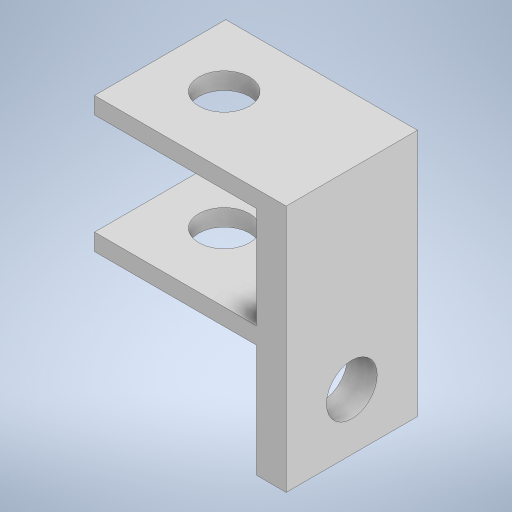
# Autodesk Inventor part: rodclamp1
Saved by Autodesk Inventor 2024.1 (Build 281209000, 209)
## iProperties
Created: 2024-01-24
Part Number: rodclamp1
Material: Generic
Document SubType Name: Modeling
Designer: udayk
Density: 1 g/cm^3
Appearance: Default
Author: udayk
Autodesk Inventor part; units mm, degrees
ref_plane "YZ Plane" through (0, 0, 0) normal (1, 0, 0) x (0, 1, 0)
ref_plane "XZ Plane" through (0, 0, 0) normal (0, 1, 0) x (-1, 0, 0)
ref_plane "XY Plane" through (0, 0, 0) normal (0, 0, 1) x (1, 0, 0)
sketch "Sketch1" plane through (0, 0, 0) normal (1, 0, 0) x (0, 1, 0)
  line L0 (0, 0) -> (12, 0)
  line L1 (12, 0) -> (12, -11.65)
  line L2 (12, -11.65) -> (0, -11.65)
  line L3 (0, -11.65) -> (0, 0)
  dimension "d0" = 12
  dimension "d1" = 11.65
  constraints: 8 end point, 2 parallel, 1 horizontal, 1 perpendicular
  measures "d0" distance of L1.end L2.end
  measures "d1" distance between parallel lines of L0 L2
extrude "Extrusion1" add sketch "Sketch1" along normal blind 17
sketch "Sketch3" plane through (0, 0, 0) normal (0, 0, 1) x (1, 0, 0)
  line L0 (-0.6451, 10.5) -> (14.3549, 10.5)
  line L1 (14.3549, 10.5) -> (14.3549, 1.5)
  line L2 (14.3549, 1.5) -> (-0.6451, 1.5)
  line L3 (-0.6451, 1.5) -> (-0.6451, 10.5)
  line L4 (17, 12) -> (17, 0) projected
  line L5 (0, 12) -> (17, 12) projected
  point P0 (0, 0)
  point P1 (10, 1.5)
  point P2 (10, 10.5)
  dimension "d7" = 9
  dimension "d8" = 15
  dimension "d10" = 1.5
  constraints: 8 end point, 2 parallel, 1 horizontal, 1 perpendicular
  measures "d7" distance between parallel lines of L2 L0
  measures "d8" distance between parallel lines of L3 L1
  measures "d10" distance between parallel lines of L5 L0
extrude "Extrusion2" cut sketch "Sketch3" against normal blind 14
sketch "Sketch5" plane through (0, 12, 0) normal (0, 1, 0) x (1, 0, 0)
  circle A0 centre (5.4549, 6.05) radius 2.25
  line L0 (14.3549, 0) -> (14.3549, 11.65) projected
  line L1 (0, 11.65) -> (17, 11.65) projected
  point P0 (0, 0)
  point P1 (11.3549, 10)
  point P2 (14.3549, 11.65)
  dimension "d16" = 4.5
  dimension "d17" = 8.9
  dimension "d18" = 5.6
  constraints: 1 centre point, 1 other
  measures "d16" diameter of A0
  measures "d18" distance from line of L1 A0.centre
extrude "Extrusion3" cut sketch "Sketch5" against normal blind 14
sketch "Sketch6" plane through (0, 0, -11.65) normal (0, -1, 0) x (1, 0, 0)
  line L0 (14.3549, 11.65) -> (14.3549, 0) projected
  line L1 (17, 11.65) -> (17, 0) projected
  line L2 (14.3549, 11.65) -> (17, 11.65)
  line L3 (17, 11.65) -> (17, 0)
  line L4 (17, 0) -> (14.3549, 0)
  line L5 (14.3549, 0) -> (14.3549, 11.65)
  point P0 (0, 11.65)
  constraints: 8 end point, 2 parallel, 1 horizontal, 1 perpendicular
extrude "Extrusion4" add sketch "Sketch6" along normal blind 10
sketch "Sketch7" plane through (14.3549, 0, -11.65) normal (-1, 0, 0) x (0, 0, 1)
  circle A0 centre (5.825, -5) radius 2.25
  line L0 (11.65, 0) -> (11.65, -10) projected
  line L1 (11.65, -10) -> (0, -10) projected
  dimension "d23" = 5.825
  dimension "d24" = 4.5
  dimension "d25" = 5
  constraints: 1 centre point
  measures "d23" distance from line of L0 A0.centre
  measures "d24" diameter of A0
  measures "d25" distance from line of L1 A0.centre
extrude "Extrusion5" cut sketch "Sketch7" against normal blind 4
body "Solid1"
